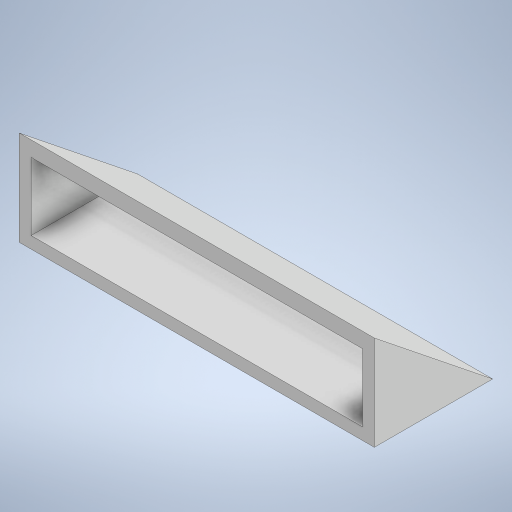
# Autodesk Inventor part: sumo_module_shield
Saved by Autodesk Inventor 2023 (Build 270158000, 158)
## iProperties
Created: 2024-04-04
Part Number: sumo_module_shield
Material: Ogólny
Document SubType Name: Modeling
Designer: Kamil
Density: 1 g/cm^3
Appearance: Domyślna
Author: Kamil
Autodesk Inventor part; units mm, degrees
ref_plane "YZ Plane" through (0, 0, 0) normal (1, 0, 0) x (0, 1, 0)
ref_plane "XZ Plane" through (0, 0, 0) normal (0, 1, 0) x (-1, 0, 0)
ref_plane "XY Plane" through (0, 0, 0) normal (0, 0, 1) x (1, 0, 0)
sketch "Szkic1" plane through (0, 0, 0) normal (1, 0, 0) x (0, 1, 0)
  line L0 (10, 15) -> (-30, 15)
  line L1 (-30, 15) -> (-30, -35)
  line L2 (-30, -35) -> (10, 15)
  point P0 (0, 0)
  dimension "d0" = 40
  dimension "d1" = 50
  constraints: 6 end point, 1 horizontal, 1 perpendicular
  measures "d0" distance of L0.start L0.end
  measures "d1" distance of L0.end L1.end
extrude "Wyciągnięcie proste1" add sketch "Szkic1" along normal blind 150
shell "Skorupa2" thickness 5 removed faces 1 at (50, -3.3333, 15)
